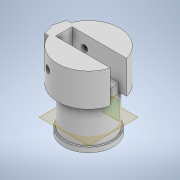
# Autodesk Inventor part: handle_base
Saved by Autodesk Inventor 2021 (Build 250183000, 183)
## iProperties
Created: 2021-03-06
Part Number: handle_base
Material: Generic
Document SubType Name: Modeling
Designer: ben
Density: 1 g/cm^3
Appearance: Default
Mass: 226.368 g
Surface Area: 425.082 cm^2
Volume: 226.368 cm^3
Author: ben
Autodesk Inventor part; units mm, degrees
ref_plane "YZ Plane" through (0, 0, 0) normal (1, 0, 0) x (0, 1, 0)
ref_plane "XZ Plane" through (0, 0, 0) normal (0, 1, 0) x (-1, 0, 0)
ref_plane "XY Plane" through (0, 0, 0) normal (0, 0, 1) x (1, 0, 0)
ref_plane "Work Plane1" through (-35, 22.5, -35) normal (0, 0, 1) x (1, 0, 0)
sketch "Sketch1" plane through (-35, 22.5, -35) normal (0, 0, 1) x (1, 0, 0)
  circle A0 centre (35, -42) radius 28
  circle A1 centre (35, -42) radius 6
  dimension "d0" = 56
  dimension "d24" = 12
  constraints: 2 centre point, 1 coincident, 1 other
  measures "d0" diameter of A0
  measures "d24" diameter of A1
ref_plane "Work Plane2" through (0, -19.5, 0) normal (0, 0, 1) x (1, 0, 0)
sketch "Sketch2" plane through (0, -19.5, 0) normal (0, 0, 1) x (1, 0, 0)
  arc A0 (-36.1421, -10) -> (-36.1421, 10) centre (0, 0) ccw
  line L0 (29.9857, -10) -> (-36.1421, -10)
  line L1 (-36.1421, 10) -> (29.9857, 10)
  line L2 (29.9857, 10) -> (29.9857, -10)
  line L3 (34.9857, -13.5) -> (39.9857, -13.5)
  line L4 (39.9857, -13.5) -> (39.9857, 13.5)
  line L5 (39.9857, 13.5) -> (34.9857, 13.5)
  line L6 (34.9857, 13.5) -> (34.9857, -13.5)
  line L7 (39.9857, -13.5) -> (43.6938, 0)
  line L8 (43.6938, 0) -> (39.9857, 13.5)
  point P0 (0, 19.5)
  point P1 (37.5, 0)
  point P2 (36.1421, 10)
  point P3 (36.1421, -10)
  dimension "d3" = 75
  dimension "d40" = 5
  dimension "d41" = 27
  dimension "d44" = 14
  dimension "d110" = 5
  constraints: 18 end point, 4 horizontal, 4 point on circle, 3 parallel, 1 centre point, 1 perpendicular, 1 vertical, 1 other
  measures "d3" diameter of A0
  measures "d40" distance of L3.start L3.end
  measures "d41" distance of L5.end L3.start
  measures "d44" distance of L3.end L7.end
  measures "d110" distance between parallel lines of L2 L6
extrude "Extrusion2" add sketch "Sketch2" along normal blind 40
ref_plane "Work Plane3" through (-36.1421, -9.5, 0) normal (0, -1, 0) x (1, 0, 0)
sketch "Sketch4" plane through (-36.1421, -9.5, 0) normal (0, -1, 0) x (1, 0, 0)
  line L0 (0, 0) -> (10.5247, 0) projected
  line L1 (0, 0) -> (66.1278, 0) projected
  line L2 (66.1278, 0) -> (66.1278, 40) projected
  line L3 (0, 40) -> (66.1278, 40) projected
  line L4 (0, 0) -> (0, 40) projected
  line L5 (0, 10) -> (66.1278, 10)
  line L6 (66.1278, 0) -> (66.1278, 40) projected
  point P0 (36.1421, 0)
  point P1 (51.1278, 25)
  dimension "d99" = 15
  dimension "d100" = 10
  dimension "d101" = 15
  constraints: 2 end point, 2 point on line, 1 horizontal
  measures "d99" distance from line of L2 point (51.128, 25)
  measures "d100" distance between parallel lines of L1 L5
  measures "d101" distance from line of L5 point (51.128, 25)
hole "Hole2" at (14.9857, -9.5, 25) direction (0, 1, 0) diameter 7.7 end through all both
extrude "Extrusion3" add sketch "Sketch1" along normal blind 35 and the other way blind 10 separate body
sketch "Sketch8" plane through (0, -19.5, -45) normal (0, 0, -1) x (-1, 0, 0)
  circle A0 centre (0, 0) radius 6 projected
  circle A1 centre (0, 0) radius 6 projected
  circle A2 centre (0, 0) radius 28 projected
  circle A3 centre (0, 0) radius 30
  line L0 (-6, 10.3923) -> (12, 0)
  line L1 (12, 0) -> (-6, -10.3923)
  line L2 (-6, -10.3923) -> (-6, 10.3923)
  point P0 (0, 19.5)
  point P1 (-6, 0)
  dimension "d107" = 2
  constraints: 6 end point, 2 coincident, 1 centre point, 1 horizontal alignment, 1 midpoint, 8 other
  measures "d107" radial gap between concentric circles of A2 A3
ref_plane "Work Plane4" through (-35, 22.5, 0) normal (0, 0, 1) x (1, 0, 0)
sketch "Sketch15" plane through (0, -19.5, 0) normal (0, 0, -1) x (-1, 0, 0)
  line L0 (36.1421, 10) -> (-29.9857, 10) projected
  circle A0 centre (0, 0) radius 28 projected
  circle A1 centre (0, 0) radius 6 projected
  line L1 (36.1421, 10) -> (-29.9857, 10) projected
  line L2 (-29.9857, 10) -> (-29.9857, -10) projected
  line L3 (-29.9857, -10) -> (36.1421, -10) projected
  arc A2 (-34.9857, -13.5) -> (36.1421, -10) centre (0, 0) ccw projected
  line L4 (-34.9857, -13.5) -> (-39.9857, -13.5) projected
  line L5 (-39.9857, -13.5) -> (-43.6938, 0) projected
  line L6 (-43.6938, 0) -> (-39.9857, 13.5) projected
  line L7 (-39.9857, 13.5) -> (-34.9857, 13.5) projected
  arc A3 (36.1421, 10) -> (-34.9857, 13.5) centre (0, 0) ccw projected
  point P0 (0, 19.5)
  point P1 (10, -10)
  point P2 (-10, -10)
  point P3 (10, 10)
  point P4 (-10, 10)
  point P5 (-26.1534, -10)
  point P6 (26.1534, -10)
  point P7 (26.1534, 10)
  point P8 (-26.1534, 10)
extrude "Extrusion12" add sketch "Sketch15" against normal blind 10 contours A0 L3 L0 bodies 2
extrude "Extrusion13" add sketch "Sketch8" along normal blind 6 contours A2 | A3 bodies 2
ref_plane "Work Plane5" through (0, -19.5, -35) normal (0, 0, 1) x (1, 0, 0)
sketch "Sketch16" plane through (0, -19.5, -35) normal (0, 0, 1) x (1, 0, 0)
  circle A0 centre (0, 0) radius 4
  circle A1 centre (0, 0) radius 6
  point P0 (0, 19.5)
  dimension "d112" = 8
  constraints: 2 centre point, 2 coincident
  measures "d112" diameter of A0
extrude "Extrusion14" add sketch "Sketch16" against normal blind 8 bodies 2
sketch "Sketch18" plane through (-35, 22.5, 0) normal (0, 0, 1) x (1, 0, 0)
  arc A0 (8.8466, -32) -> (8.8466, -52) centre (35, -42) ccw projected
  line L0 (8.8466, -52) -> (61.1534, -52) projected
  arc A1 (61.1534, -52) -> (61.1534, -32) centre (35, -42) ccw projected
  line L1 (61.1534, -32) -> (8.8466, -32) projected
  circle A2 centre (35, -42) radius 6 projected
  line L2 (41, -48) -> (29, -48)
  line L3 (29, -48) -> (29, -56)
  line L4 (29, -56) -> (41, -56)
  line L5 (41, -56) -> (41, -48)
  line L6 (61.1534, -52) -> (8.8466, -52) projected
  line L7 (41, -48) -> (29, -56) construction
  line L8 (29, -48) -> (41, -56) construction
  line L9 (41, -28) -> (29, -28)
  line L10 (29, -28) -> (29, -36)
  line L11 (29, -36) -> (41, -36)
  line L12 (41, -36) -> (41, -28)
  line L13 (8.8466, -32) -> (61.1534, -32) projected
  line L14 (41, -28) -> (29, -36) construction
  line L15 (29, -28) -> (41, -36) construction
  point P0 (35, -52)
  point P1 (35, -32)
  point P2 (41, -52)
  point P3 (29, -52)
  point P4 (29, -32)
  point P5 (41, -32)
  dimension "d120" = 12
  dimension "d121" = 8
  dimension "d122" = 12
  dimension "d123" = 8
  constraints: 24 end point, 6 midpoint, 4 parallel, 2 horizontal, 2 perpendicular
  measures "d120" distance of L4.end L3.end
  measures "d121" distance of L3.end L2.end
  measures "d122" distance of L11.end L10.end
  measures "d123" distance of L10.end L9.end
extrude "Extrusion15" add sketch "Sketch18" along normal blind 8 contours L10 L9 L12 L1 | L0 L5 L4 L3 bodies 2
sketch "Sketch19" plane through (0, -19.5, 0) normal (0, 0, -1) x (-1, 0, 0)
  arc A0 (26.1534, -10) -> (26.1534, 10) centre (0, 0) ccw projected
  line L0 (26.1534, -10) -> (-26.1534, -10) projected
  arc A1 (-26.1534, 10) -> (-26.1534, -10) centre (0, 0) ccw projected
  line L1 (-26.1534, 10) -> (26.1534, 10) projected
  circle A2 centre (0, 0) radius 6 projected
  line L2 (-6, 10) -> (6, 10)
  line L3 (36.1421, 10) -> (-29.9857, 10) projected
  line L4 (6, -10) -> (-6, -10)
  line L5 (-29.9857, -10) -> (36.1421, -10) projected
  line L6 (6, 5.8) -> (-6, 5.8)
  line L7 (-6, 5.8) -> (-6, 14.2)
  line L8 (-6, 14.2) -> (6, 14.2)
  line L9 (6, 14.2) -> (6, 5.8)
  line L10 (6, 5.8) -> (-6, 14.2) construction
  line L11 (-6, 5.8) -> (6, 14.2) construction
  line L12 (-6, -5.8) -> (6, -5.8)
  line L13 (6, -5.8) -> (6, -14.2)
  line L14 (6, -14.2) -> (-6, -14.2)
  line L15 (-6, -14.2) -> (-6, -5.8)
  line L16 (-29.9857, -10) -> (36.1421, -10) projected
  line L17 (-6, -5.8) -> (6, -14.2) construction
  line L18 (6, -5.8) -> (-6, -14.2) construction
  point P0 (0, 19.5)
  point P1 (0, 10)
  point P2 (0, -10)
  dimension "d128" = 12
  dimension "d129" = 8.4
  dimension "d130" = 12
  dimension "d131" = 8.4
  constraints: 28 end point, 4 midpoint, 4 parallel, 2 collinear, 2 horizontal, 2 perpendicular, 2 point on line
  measures "d128" distance of L7.end L8.end
  measures "d129" distance of L6.end L7.end
  measures "d130" distance of L13.end L14.end
  measures "d131" distance of L12.end L13.end
extrude "Extrusion16" cut sketch "Sketch19" against normal blind 8 contours L13 L14 L15 L0 | L1 L7 L8 L9 bodies 1
equation "\"d113\" = d112"
